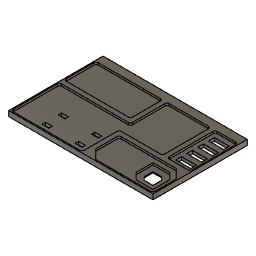
Door (Autodesk Fusion 360 archive; units mm, degrees)
design "Lower Interface (v5)"
Autodesk Fusion 360 part; units mm, degrees
sketch "Sketch1" plane through (0, 0, 0) normal (0, 0, 1) x (1, 0, 0)
  line L0 (0, 0) -> (70.4, 0)
  line L1 (70.4, 0) -> (70.4, 46.4)
  line L2 (70.4, 46.4) -> (0, 46.4)
  line L3 (0, 46.4) -> (0, 0)
  line L4 (1.1, 1.1) -> (69.3, 1.1) construction
  line L5 (69.3, 1.1) -> (69.3, 45.3) construction
  line L6 (69.3, 45.3) -> (1.1, 45.3) construction
  line L7 (1.1, 45.3) -> (1.1, 1.1) construction
  line L8 (35.2, 45.3) -> (35.2, 1.1) construction
  line L9 (1.1, 23.2) -> (35.2, 23.2) construction
  line L10 (35.2, 23.2) -> (69.3, 23.2) construction
  line L11 (35.2, 45.3) -> (35.2, 42) construction
  line L12 (35.2, 42) -> (35, 42) construction
  line L13 (35, 42) -> (1.1, 42) construction
  line L14 (35.2, 42) -> (69.3, 42) construction
  line L15 (68.3, 42) -> (59.3, 42)
  line L16 (58.3, 41) -> (58.3, 19.9)
  line L17 (59.3, 18.9) -> (68.3, 18.9)
  line L18 (69.3, 19.9) -> (69.3, 41)
  line L19 (58.3, 30.45) -> (56.1, 30.45) construction
  line L20 (36.2, 42) -> (55.1, 42)
  line L21 (56.1, 41) -> (56.1, 19.9)
  line L22 (55.1, 18.9) -> (36.2, 18.9)
  line L23 (35.2, 30.45) -> (33, 30.45) construction
  line L24 (2.1, 42) -> (32, 42)
  line L25 (33, 41) -> (33, 27.6)
  line L26 (32, 26.6) -> (2.1, 26.6)
  line L27 (1.1, 27.6) -> (1.1, 41)
  line L28 (17.05, 26.6) -> (17.05, 24.4) construction
  line L29 (45.65, 18.9) -> (45.65, 16.7) construction
  line L30 (2.1, 1.1) -> (34.2, 1.1)
  line L31 (34.2, 24.3632) -> (2.1, 24.3632)
  line L32 (1.1, 23.3632) -> (1.1, 2.1)
  line L33 (35.2, 41) -> (35.2, 25.3632)
  line L34 (35.2, 17.9) -> (35.2, 2.1)
  line L35 (18.15, 24.3632) -> (18.15, 17.7632) construction
  line L36 (1.1, 1.1) -> (1.1, 2.2) construction
  line L37 (1.1, 1.1) -> (2.2, 1.1) construction
  line L38 (35.2, 1.1) -> (35.2, 2.2) construction
  line L39 (35.2, 1.1) -> (34.1, 1.1) construction
  line L40 (2.2, 2.2) -> (34.1, 2.2) construction
  line L41 (34.1, 2.2) -> (34.1, 17.7632) construction
  line L42 (34.1, 17.7632) -> (18.15, 17.7632) construction
  line L43 (2.2, 2.2) -> (2.2, 17.7632) construction
  line L44 (2.2, 17.7632) -> (18.15, 17.7632) construction
  line L45 (18.15, 2.2) -> (18.15, 17.7632) construction
  line L46 (18.15, 9.9816) -> (34.1, 9.9816) construction
  line L47 (18.15, 9.9816) -> (2.2, 9.9816) construction
  line L48 (10.175, 9.9816) -> (10.175, 11.0816) construction
  line L49 (18.15, 9.9816) -> (18.15, 17.7632) construction
  line L50 (18.15, 9.9816) -> (18.15, 2.2) construction
  line L51 (18.15, 13.8724) -> (17.05, 13.8724) construction
  line L52 (2.2, 2.2) -> (18.15, 2.2) construction
  line L53 (18.15, 2.2) -> (34.1, 2.2) construction
  line L54 (10.175, 2.2) -> (10.175, 3.3) construction
  line L55 (18.15, 6.0908) -> (17.05, 6.0908) construction
  line L56 (26.125, 2.2) -> (26.125, 3.3) construction
  line L57 (18.15, 6.0908) -> (19.25, 6.0908) construction
  line L58 (18.15, 13.8724) -> (19.25, 13.8724) construction
  line L59 (26.125, 9.9816) -> (26.125, 11.0816) construction
  line L60 (3.3, 16.6632) -> (17.05, 16.6632) construction
  line L61 (17.05, 16.6632) -> (17.05, 11.0816) construction
  line L62 (17.05, 11.0816) -> (3.3, 11.0816) construction
  line L63 (3.3, 11.0816) -> (3.3, 16.6632) construction
  line L64 (3.3, 8.8816) -> (17.05, 8.8816) construction
  line L65 (17.05, 8.8816) -> (17.05, 3.3) construction
  line L66 (17.05, 3.3) -> (3.3, 3.3) construction
  line L67 (3.3, 3.3) -> (3.3, 8.8816) construction
  line L68 (19.25, 8.8816) -> (33, 8.8816) construction
  line L69 (33, 8.8816) -> (33, 3.3) construction
  line L70 (33, 3.3) -> (19.25, 3.3) construction
  line L71 (19.25, 3.3) -> (19.25, 8.8816) construction
  line L72 (19.25, 16.6632) -> (33, 16.6632) construction
  line L73 (33, 16.6632) -> (33, 11.0816) construction
  line L74 (33, 11.0816) -> (19.25, 11.0816) construction
  line L75 (19.25, 11.0816) -> (19.25, 16.6632) construction
  line L76 (17.05, 11.0816) -> (17.05, 11.6316) construction
  line L77 (17.05, 11.0816) -> (16.5, 11.0816) construction
  line L78 (33, 11.0816) -> (33, 11.6316) construction
  line L79 (33, 11.0816) -> (32.45, 11.0816) construction
  line L80 (33, 3.3) -> (33, 3.85) construction
  line L81 (33, 3.3) -> (32.45, 3.3) construction
  line L82 (17.05, 3.3) -> (16.5, 3.3) construction
  line L83 (17.05, 3.3) -> (17.05, 3.85) construction
  line L84 (16.5, 11.6316) -> (13.2, 11.6316)
  line L85 (13.2, 11.6316) -> (13.2, 13.2816)
  line L86 (13.2, 13.2816) -> (16.5, 13.2816)
  line L87 (16.5, 13.2816) -> (16.5, 11.6316)
  line L88 (32.45, 11.6316) -> (29.15, 11.6316)
  line L89 (29.15, 11.6316) -> (29.15, 13.2816)
  line L90 (29.15, 13.2816) -> (32.45, 13.2816)
  line L91 (32.45, 13.2816) -> (32.45, 11.6316)
  line L92 (32.45, 3.85) -> (29.15, 3.85)
  line L93 (29.15, 3.85) -> (29.15, 5.5)
  line L94 (29.15, 5.5) -> (32.45, 5.5)
  line L95 (32.45, 5.5) -> (32.45, 3.85)
  line L96 (16.5, 3.85) -> (13.2, 3.85)
  line L97 (13.2, 3.85) -> (13.2, 5.5)
  line L98 (13.2, 5.5) -> (16.5, 5.5)
  line L99 (16.5, 5.5) -> (16.5, 3.85)
  line L100 (35.2, 10) -> (37.4, 10) construction
  line L101 (37.4, 16.7) -> (69.3, 16.7) construction
  line L102 (69.3, 16.7) -> (64.9, 16.7) construction
  line L103 (69.3, 16.7) -> (69.3, 12.3) construction
  line L104 (64.9, 16.7) -> (69.3, 12.3)
  line L105 (37.4, 1.1) -> (37.4, 5.5) construction
  line L106 (37.4, 1.1) -> (41.8, 1.1) construction
  line L107 (37.4, 5.5) -> (41.8, 1.1)
  line L108 (37.4, 15.7) -> (37.4, 5.5)
  line L109 (38.4, 16.7) -> (64.9, 16.7)
  line L110 (69.3, 12.3) -> (69.3, 2.1)
  line L111 (68.3, 1.1) -> (41.8, 1.1)
  line L112 (67.1, 14.5) -> (65.5444, 12.9444) construction
  line L113 (65.5444, 12.9444) -> (67.1, 11.3887)
  line L114 (65.5444, 12.9444) -> (63.9887, 14.5)
  line L115 (67.1, 11.3887) -> (69.3, 11.4) construction
  line L116 (63.9887, 14.5) -> (64, 16.7) construction
  line L117 (67.1, 1.1) -> (67.1, 3.3) construction
  line L118 (67.1, 11.3887) -> (67.1, 3.3)
  line L119 (67.1, 3.3) -> (59.011, 3.3)
  line L120 (63.9887, 14.5) -> (55.8998, 14.5414)
  line L121 (55.8998, 14.5414) -> (55.8584, 6.4525)
  line L122 (55.8584, 6.4525) -> (59.011, 3.3)
  line L123 (58.6142, 7.5858) -> (60.1501, 6.05)
  line L124 (64.35, 6.05) -> (60.1501, 6.05)
  line L125 (64.35, 10.2496) -> (64.35, 6.05)
  line L126 (63.5998, 10.9998) -> (64.35, 10.2496)
  line L127 (63.5998, 10.9998) -> (62.8438, 11.7558)
  line L128 (62.8438, 11.7558) -> (58.6357, 11.7774)
  line L129 (58.6357, 11.7774) -> (58.6142, 7.5858)
  arc A0 (2.1, 42) -> (1.1, 41) centre (2.1, 41) ccw
  arc A1 (33, 41) -> (32, 42) centre (32, 41) ccw
  arc A2 (32, 26.6) -> (33, 27.6) centre (32, 27.6) ccw
  arc A3 (1.1, 27.6) -> (2.1, 26.6) centre (2.1, 27.6) ccw
  arc A4 (36.2, 42) -> (35.2, 41) centre (36.2, 41) ccw
  arc A5 (56.1, 41) -> (55.1, 42) centre (55.1, 41) ccw
  arc A6 (55.1, 18.9) -> (56.1, 19.9) centre (55.1, 19.9) ccw
  arc A7 (36.2, 18.9) -> (35.2, 17.9) centre (36.2, 17.9) ccw
  arc A8 (34.2, 1.1) -> (35.2, 2.1) centre (34.2, 2.1) ccw
  arc A9 (1.1, 2.1) -> (2.1, 1.1) centre (2.1, 2.1) ccw
  arc A10 (2.1, 24.3632) -> (1.1, 23.3632) centre (2.1, 23.3632) ccw
  arc A11 (34.2, 24.3632) -> (35.2, 25.3632) centre (34.2, 25.3632) ccw
  arc A12 (38.4, 16.7) -> (37.4, 15.7) centre (38.4, 15.7) ccw
  arc A13 (68.3, 1.1) -> (69.3, 2.1) centre (68.3, 2.1) ccw
  arc A14 (59.3, 42) -> (58.3, 41) centre (59.3, 41) ccw
  arc A15 (58.3, 19.9) -> (59.3, 18.9) centre (59.3, 19.9) ccw
  arc A16 (68.3, 18.9) -> (69.3, 19.9) centre (68.3, 19.9) ccw
  arc A17 (69.3, 41) -> (68.3, 42) centre (68.3, 41) ccw
  line L130 (58.3, 41) -> (69.3, 41) construction
  line L131 (58.3, 19.9) -> (69.3, 19.9) construction
  line L132 (63.8, 19.9) -> (63.8, 41) construction
  line L133 (60.225, 39.7375) -> (67.375, 39.7375)
  line L134 (67.375, 39.7375) -> (67.375, 36.9875)
  line L135 (67.375, 36.9875) -> (60.225, 36.9875)
  line L136 (60.225, 36.9875) -> (60.225, 39.7375)
  line L137 (63.8, 41) -> (63.8, 39.7375) construction
  line L138 (60.225, 31.7115) -> (60.225, 34.4615)
  line L139 (60.225, 34.4615) -> (67.375, 34.4615)
  line L140 (67.375, 31.7115) -> (60.225, 31.7115)
  line L141 (67.375, 34.4615) -> (67.375, 31.7115)
  line L142 (67.375, 26.4355) -> (60.225, 26.4355)
  line L143 (60.225, 26.4355) -> (60.225, 29.1855)
  line L144 (67.375, 29.1855) -> (67.375, 26.4355)
  line L145 (60.225, 29.1855) -> (67.375, 29.1855)
  line L146 (60.225, 21.1595) -> (60.225, 23.9095)
  line L147 (60.225, 23.9095) -> (67.375, 23.9095)
  line L148 (67.375, 21.1595) -> (60.225, 21.1595)
  line L149 (67.375, 23.9095) -> (67.375, 21.1595)
  line L150 (63.8, 36.9875) -> (63.8, 34.4615) construction
  line L151 (63.8, 31.7115) -> (63.8, 29.1855) construction
  line L152 (63.8, 26.4355) -> (63.8, 23.9095) construction
  line L153 (70.4, 33.0328) -> (68.4, 33.0328) construction
  line L154 (13.2, 4.675) -> (11.2, 4.675) construction
  line L155 (14.85, 3.85) -> (14.85, 1.85) construction
  line L156 (11.2, 1.85) -> (68.3, 1.85)
  line L157 (68.3, 1.85) -> (68.3, 42.6341)
  line L158 (68.3, 42.6341) -> (11.2, 42.6341)
  line L159 (11.2, 42.6341) -> (11.2, 1.85)
  point P0 (58.3, 42)
  point P1 (69.3, 18.9)
  point P2 (56.1, 42)
  point P3 (56.1, 18.9)
  point P4 (35.2, 18.9)
  point P5 (1.1, 26.6)
  dimension "d1" = 46.4
  dimension "d2" = 70.4
  dimension "d3" = -1.1
  dimension "d5" = 3.3
  dimension "d6" = 11
  dimension "d7" = 23.1
  dimension "d8" = 2.2
  dimension "d9" = 23.1
  dimension "d10" = 20.9
  dimension "d11" = 2.2
  dimension "d12" = 15.4
  dimension "d13" = 2.2
  dimension "d14" = 2.2
  dimension "d16" = 6.6
  dimension "d18" = 1.1
  dimension "d19" = 1.1
  dimension "d20" = 1.1
  dimension "d21" = 1.1
  dimension "d22" = 1.1
  dimension "d23" = 1.1
  dimension "d24" = 1.1
  dimension "d25" = 1.1
  dimension "d26" = 1.1
  dimension "d27" = 1.1
  dimension "d28" = 1.1
  dimension "d29" = 1.1
  dimension "d30" = 0.55
  dimension "d31" = 0.55
  dimension "d32" = 0.55
  dimension "d33" = 0.55
  dimension "d34" = 0.55
  dimension "d35" = 0.55
  dimension "d36" = 0.55
  dimension "d37" = 0.55
  dimension "d38" = 3.3
  dimension "d39" = 1.65
  dimension "d40" = 3.3
  dimension "d41" = 1.65
  dimension "d42" = 3.3
  dimension "d43" = 1.65
  dimension "d44" = 3.3
  dimension "d45" = 1.65
  dimension "d46" = 2.2
  dimension "d47" = 4.4
  dimension "d48" = 4.4
  dimension "d49" = 4.4
  dimension "d50" = 4.4
  dimension "d51" = 2.2
  dimension "d52" = 2.2
  dimension "d53" = 2.2
  dimension "d55" = 2.2
  dimension "d56" = 8.089
  dimension "d57" = 8.089
  dimension "d58" = 8.089
  dimension "d59" = -2.75
  dimension "d60" = 1
  dimension "d61" = 1
  dimension "d62" = 1
  dimension "d63" = 1
  dimension "d64" = 1
  dimension "d65" = 2.75
  dimension "d66" = 1.2625
  dimension "d67" = 7.15
  dimension "d68" = 2.75
  dimension "d69" = 7.15
  dimension "d70" = 2.75
  dimension "d71" = 7.15
  dimension "d72" = 2.75
  dimension "d73" = 7.15
  dimension "d74" = 2.526
  dimension "d75" = 2.526
  dimension "d76" = 2.526
  dimension "d93" = 2
  dimension "d94" = 2
  dimension "d95" = 2
  constraint horizontal L0
  constraint vertical L1
  constraint horizontal L2
  constraint vertical L3
  constraint coincident L0.start L3.end
  constraint midpoint L6 L8.start
  constraint midpoint L4 L8.end
  constraint midpoint L7 L9.start
  constraint midpoint L8 L9.end
  constraint midpoint L5 L10.end
  constraint perpendicular L6 L11
  constraint perpendicular L11 L12
  constraint coincident L7 L13.end
  constraint perpendicular L7 L13
  constraint coincident L5 L14.end
  constraint perpendicular L5 L14
  constraint horizontal L15
  constraint vertical L16
  constraint horizontal L17
  constraint vertical L18
  constraint perpendicular L16 L19
  constraint horizontal L20
  constraint vertical L21
  constraint horizontal L22
  constraint horizontal L24
  constraint vertical L25
  constraint horizontal L26
  constraint vertical L27
  constraint perpendicular L26 L28
  constraint perpendicular L22 L29
  constraint horizontal L30
  constraint horizontal L31
  constraint vertical L32
  constraint perpendicular L23 L33
  constraint perpendicular L30 L34
  constraint perpendicular L9 L35
  constraint perpendicular L30 L36
  constraint perpendicular L7 L37
  constraint perpendicular L4 L38
  constraint perpendicular L38 L39
  constraint perpendicular L8 L40
  constraint perpendicular L40 L41
  constraint perpendicular L35 L42
  constraint perpendicular L42 L43
  constraint perpendicular L35 L44
  constraint midpoint L40 L45.start
  constraint perpendicular L44 L45
  constraint midpoint L45 L46.start
  constraint midpoint L41 L46.end
  constraint midpoint L43 L47.end
  constraint midpoint L47 L48.start
  constraint perpendicular L47 L48
  constraint midpoint L49 L51.start
  constraint perpendicular L45 L51
  constraint midpoint L52 L54.start
  constraint perpendicular L52 L54
  constraint midpoint L50 L55.start
  constraint perpendicular L50 L55
  constraint midpoint L53 L56.start
  constraint perpendicular L53 L56
  constraint perpendicular L45 L57
  constraint perpendicular L45 L58
  constraint midpoint L46 L59.start
  constraint perpendicular L46 L59
  constraint horizontal L60
  constraint vertical L61
  constraint horizontal L62
  constraint vertical L63
  constraint horizontal L64
  constraint vertical L65
  constraint horizontal L66
  constraint vertical L67
  constraint horizontal L68
  constraint vertical L69
  constraint horizontal L70
  constraint vertical L71
  constraint horizontal L72
  constraint vertical L73
  constraint horizontal L74
  constraint vertical L75
  constraint midpoint L48.end L62
  constraint midpoint L51.end L61
  constraint midpoint L54.end L66
  constraint midpoint L55.end L65
  constraint midpoint L56.end L70
  constraint midpoint L57.end L71
  constraint midpoint L58.end L75
  constraint midpoint L59.end L74
  constraint perpendicular L62 L76
  constraint perpendicular L76 L77
  constraint perpendicular L74 L78
  constraint perpendicular L78 L79
  constraint perpendicular L70 L80
  constraint perpendicular L69 L81
  constraint perpendicular L65 L82
  constraint perpendicular L82 L83
  constraint horizontal L84
  constraint vertical L85
  constraint horizontal L86
  constraint vertical L87
  constraint horizontal L88
  constraint vertical L89
  constraint horizontal L90
  constraint vertical L91
  constraint horizontal L92
  constraint vertical L93
  constraint horizontal L94
  constraint vertical L95
  constraint horizontal L96
  constraint vertical L97
  constraint horizontal L98
  constraint vertical L99
  constraint perpendicular L34 L100
  constraint horizontal L101
  constraint perpendicular L101 L103
  constraint perpendicular L105 L106
  constraint perpendicular L100 L108
  constraint perpendicular L108 L109
  constraint perpendicular L4 L110
  constraint perpendicular L110 L111
  constraint midpoint L104 L112.start
  constraint perpendicular L104 L112
  constraint perpendicular L112 L113
  constraint perpendicular L112 L114
  constraint coincident L110 L115.end
  constraint coincident L101 L116.end
  constraint coincident L111 L117.start
  constraint perpendicular L111 L117
  constraint parallel L117 L118
  constraint perpendicular L117 L119
  constraint perpendicular L116 L120
  constraint perpendicular L120 L121
  constraint coincident L13.end L27
  constraint coincident L13.end L24
  constraint tangent L27 A0
  constraint tangent L24 A0
  constraint tangent L24 A1
  constraint tangent L25 A1
  constraint equal A0 A1
  constraint coincident L26 L28.start
  constraint tangent L25 A2
  constraint tangent L26 A2
  constraint equal A0 A2
  constraint coincident P5 L26
  constraint coincident P5 L27
  constraint tangent L26 A3
  constraint tangent L27 A3
  constraint equal A0 A3
  constraint tangent L33 A4
  constraint tangent L20 A4
  constraint coincident L19.end L21
  constraint coincident P2 L20
  constraint coincident P2 L21
  constraint tangent L20 A5
  constraint tangent L21 A5
  constraint equal A4 A5
  constraint coincident L22 L29.start
  constraint coincident P3 L21
  constraint coincident P3 L22
  constraint tangent L21 A6
  constraint tangent L22 A6
  constraint equal A4 A6
  constraint coincident L34 L100.start
  constraint coincident P4 L22
  constraint coincident P4 L34
  constraint tangent L22 A7
  constraint tangent L34 A7
  constraint equal A4 A7
  constraint coincident L8.end L34
  constraint coincident L8.end L30
  constraint tangent L34 A8
  constraint tangent L30 A8
  constraint equal A4 A8
  constraint coincident L4.start L30
  constraint coincident L4.start L32
  constraint tangent L30 A9
  constraint tangent L32 A9
  constraint equal A4 A9
  constraint coincident L31 L35.start
  constraint tangent L32 A10
  constraint tangent L31 A10
  constraint equal A4 A10
  constraint tangent L31 A11
  constraint tangent L33 A11
  constraint equal A4 A11
  constraint coincident L101.start L108
  constraint coincident L101.start L109
  constraint tangent L108 A12
  constraint tangent L109 A12
  constraint coincident L4.end L111
  constraint coincident L4.end L110
  constraint tangent L111 A13
  constraint tangent L110 A13
  constraint coincident L16 L19.start
  constraint coincident P0 L15
  constraint coincident P0 L16
  constraint tangent L15 A14
  constraint tangent L16 A14
  constraint tangent L16 A15
  constraint tangent L17 A15
  constraint equal A14 A15
  constraint coincident P1 L17
  constraint coincident P1 L18
  constraint tangent L17 A16
  constraint tangent L18 A16
  constraint equal A14 A16
  constraint coincident L14.end L18
  constraint coincident L14.end L15
  constraint tangent L18 A17
  constraint tangent L15 A17
  constraint equal A14 A17
  constraint perpendicular L5 L131
  constraint midpoint L131 L132.start
  constraint midpoint L130 L132.end
  constraint perpendicular L130 L132
  constraint horizontal L133
  constraint vertical L134
  constraint horizontal L135
  constraint vertical L136
  constraint perpendicular L130 L137
  constraint horizontal L139
  constraint vertical L141
  constraint horizontal L140
  constraint vertical L138
  constraint horizontal L145
  constraint vertical L144
  constraint horizontal L142
  constraint vertical L143
  constraint horizontal L147
  constraint vertical L149
  constraint horizontal L148
  constraint vertical L146
  constraint midpoint L133 L137.end
  constraint midpoint L135 L150.start
  constraint perpendicular L135 L150
  constraint midpoint L139 L150.end
  constraint midpoint L140 L151.start
  constraint perpendicular L140 L151
  constraint midpoint L145 L151.end
  constraint midpoint L142 L152.start
  constraint perpendicular L142 L152
  constraint midpoint L147 L152.end
  constraint coincident L1 L153.start
  constraint perpendicular L18 L153
  constraint midpoint L97 L154.start
  constraint perpendicular L97 L154
  constraint midpoint L96 L155.start
  constraint perpendicular L66 L155
  constraint horizontal L156
  constraint vertical L157
  constraint horizontal L158
  constraint vertical L159
  measures "d1" distance of L0.start L2.end
  measures "d2" distance of L1.end L2.end
  measures "d5" distance of L8.start L11.end
  measures "d6" distance of L14.end P0
  measures "d7" distance of L14.end P1
  measures "d8" distance of L19.start L19.end
  measures "d9" distance of P2 P3
  measures "d10" distance of P3 P4
  measures "d11" distance of L23.start L23.end
  measures "d12" distance of L13.end P5
  measures "d13" distance of L28.start L28.end
  measures "d14" distance of L29.start L29.end
  measures "d16" distance of L35.start L35.end
  measures "d18" distance of L4.start L36.end
  measures "d19" distance of L4.start L37.end
  measures "d20" distance of L8.end L38.end
  measures "d21" distance of L8.end L39.end
  measures "d22" distance of L48.start L48.end
  measures "d23" distance of L51.start L51.end
  measures "d24" distance of L54.start L54.end
  measures "d25" distance of L55.start L55.end
  measures "d26" distance of L56.start L56.end
  measures "d27" distance of L55.start L57.end
  measures "d28" distance of L51.start L58.end
  measures "d29" distance of L59.start L59.end
  measures "d30" distance of L61.end L76.end
  measures "d31" distance of L61.end L77.end
  measures "d32" distance of L73.end L78.end
  measures "d33" distance of L73.end L79.end
  measures "d34" distance of L69.end L80.end
  measures "d35" distance of L69.end L81.end
  measures "d36" distance of L65.end L82.end
  measures "d37" distance of L65.end L83.end
  measures "d38" distance of L84.start L84.end
  measures "d39" distance of L84.start L86.end
  measures "d40" distance of L88.start L88.end
  measures "d41" distance of L88.start L90.end
  measures "d42" distance of L92.start L92.end
  measures "d43" distance of L92.start L94.end
  measures "d44" distance of L96.start L96.end
  measures "d45" distance of L96.start L98.end
  measures "d46" distance of L100.start L100.end
  measures "d47" distance of L101.end L102.end
  measures "d48" distance of L101.end L103.end
  measures "d49" distance of L105.start L105.end
  measures "d50" distance of L105.start L106.end
  measures "d51" distance of L112.start L112.end
  measures "d52" distance of L112.end L113.end
  measures "d53" distance of L112.end L114.end
  measures "d55" distance of L117.start L117.end
  measures "d56" distance of L117.end L119.end
  measures "d57" distance of L114.end L120.end
  measures "d58" distance of L120.end L121.end
  measures "d60" radius of A0
  measures "d61" radius of A4
  measures "d62" radius of A12
  measures "d63" radius of A13
  measures "d64" radius of A14
  measures "d65" distance of L133.start L135.end
  measures "d66" distance of L132.end L137.end
  measures "d67" distance of L133.start L133.end
  measures "d68" distance of L138.start L138.end
  measures "d69" distance of L139.end L138.end
  measures "d70" distance of L143.end L142.end
  measures "d71" distance of L144.start L143.end
  measures "d72" distance of L146.end L146.start
  measures "d73" distance of L146.end L147.end
  measures "d74" distance of L150.start L150.end
  measures "d75" distance of L151.start L151.end
  measures "d76" distance of L152.start L152.end
  measures "d93" distance of L153.start L153.end
  measures "d94" distance of L154.start L154.end
  measures "d95" distance of L155.start L155.end
extrude "Extrude1" add sketch "Sketch1" against normal blind 2.5 contours L0 L1 L2 L3 | L15 L16 L17 A14 A15 L157 | L18 A16 A17 L157 | L15 L16 L17 L20 L21 L22 L24 L25 L26 L31 L33 L34 L104 L107 L108 L109 A1 A2 A4 A5 A6 A7 A8 A11 A12 A14 A15 L156 L157 L158 L159 | L104 L107 L108 L109 A12 L156 L157 | L104 L107 L110 L111 A13 L156 L157 | L24 L26 L27 A0 A3 L159 | L24 L25 L26 A1 A2 L159 | L20 L21 L22 L31 L33 L34 A4 A5 A6 A7 A8 A11 L156 L159 | L30 L31 L32 A8 A9 A10 L156 L159 | L84 L85 L86 L87 | L88 L89 L90 L91 | L92 L93 L94 L95 | L96 L97 L98 L99 | L113 L114 L118 L119 L120 L121 L122 | L123 L124 L125 L126 L127 L128 L129 | L133 L134 L135 L136 | L138 L139 L140 L141 | L142 L143 L144 L145 | L146 L147 L148 L149
extrude "Extrude2" cut sketch "Sketch1" against normal blind 1 contours L15 L16 L17 A14 A15 L157 | L18 A16 A17 L157 | L104 L107 L108 L109 A12 L156 L157 | L104 L107 L110 L111 A13 L156 L157 | L24 L26 L27 A0 A3 L159 | L24 L25 L26 A1 A2 L159 | L20 L21 L22 L31 L33 L34 A4 A5 A6 A7 A8 A11 L156 L159 | L30 L31 L32 A8 A9 A10 L156 L159 | L84 L85 L86 L87 | L88 L89 L90 L91 | L92 L93 L94 L95 | L96 L97 L98 L99 | L113 L114 L118 L119 L120 L121 L122 | L123 L124 L125 L126 L127 L128 L129 | L133 L134 L135 L136 | L138 L139 L140 L141 | L142 L143 L144 L145 | L146 L147 L148 L149
extrude "Extrude3" cut sketch "Sketch1" against normal blind 2 contours L113 L114 L118 L119 L120 L121 L122 | L123 L124 L125 L126 L127 L128 L129
extrude "Extrude4" cut sketch "Sketch1" against normal blind 10 contours L84 L85 L86 L87 | L88 L89 L90 L91 | L92 L93 L94 L95 | L96 L97 L98 L99 | L123 L124 L125 L126 L127 L128 L129 | L133 L134 L135 L136 | L138 L139 L140 L141 | L142 L143 L144 L145 | L146 L147 L148 L149
extrude "Extrude5" cut 1 faces at (23.4667, 0, -0.8333) along direction (0, 1, 0) blind 0.5
extrude "Extrude6" cut 1 faces at (46.9333, 46.4, -0.8333) along direction (0, -1, 0) blind 0.5
extrude "Extrude7" cut 1 faces at (70.4, 15.6333, -0.8333) along direction (-1, 0, 0) blind 0.5
extrude "Extrude8" cut 1 faces at (0, 30.7667, -0.8333) along direction (1, 0, 0) blind 0.5
